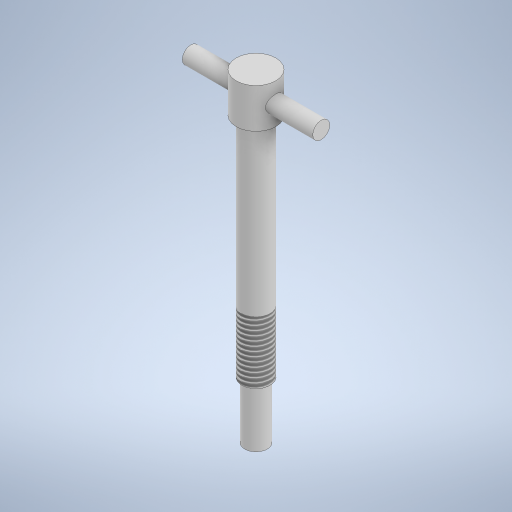
# Autodesk Inventor part: HUDSON-1-84
Saved by Autodesk Inventor 2024.2 (Build 282272000, 272)
## iProperties
Created: 2024-10-05
Part Number: HUDSON-1-84
Material: Generic
Document SubType Name: Modeling
Designer: melim
Density: 1 g/cm^3
Appearance: Default
Author: melim
Autodesk Inventor part; units mm, degrees
ref_plane "YZ Plane" through (0, 0, 0) normal (1, 0, 0) x (0, 1, 0)
ref_plane "XZ Plane" through (0, 0, 0) normal (0, 1, 0) x (-1, 0, 0)
ref_plane "XY Plane" through (0, 0, 0) normal (0, 0, 1) x (1, 0, 0)
sketch "Sketch1" plane through (0, 0, 0) normal (0, 0, 1) x (1, 0, 0)
  line L0 (-2.5, -7) -> (-2.5, -47)
  line L1 (-3.5, 0) -> (-3.5, -7)
  line L2 (-3.5, -7) -> (-2.5, -7)
  line L3 (-2, -47) -> (-2, -57)
  line L4 (-2.5, -47) -> (-2, -47)
  line L5 (-2, -57) -> (0, -57)
  line L6 (-3.5, 0) -> (0, 0)
  line L7 (0, 0) -> (0, -59)
  dimension "d1" = 7
  dimension "d3" = 40
  dimension "d5" = 10
  constraints: 17 end point, 4 horizontal, 2 vertical, 1 point on line
  measures "d1" distance of L1.start L1.end
  measures "d3" distance of L0.start L0.end
  measures "d5" distance of L3.start L3.end
revolve "Revolution1" add sketch "Sketch1" angle 360 about axis through (0, 0, 0) along (0, -1, 0)
thread "Thread1" size "M5x0.8" class "6g" standard "ANSI Metric M Profile" length 11
sketch "Sketch2" plane through (0, 0, 0) normal (1, 0, 0) x (0, 1, 0)
  line L0 (-7, 3.5) -> (-7, -3.5) projected
  line L1 (0, 3.5) -> (0, -3.5) projected
  circle A0 centre (-3.5, 0) radius 1.5
  point P0 (0, 0)
  dimension "d11" = 3
  dimension "d12" = 3.5
  dimension "d13" = 3.5
  constraints: 1 centre point
  measures "d11" diameter of A0
  measures "d12" distance from line of L1 A0.centre
  measures "d13" horizontal distance of A0.centre L0.end
extrude "Extrusion1" add sketch "Sketch2" along normal mid plane 23
body "Solid1"
